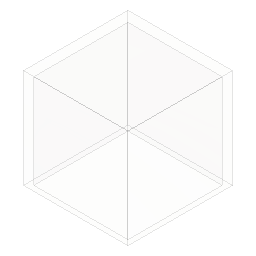
9. Sizing Box (18x18x18in) (Autodesk Fusion 360 design; units mm, degrees)
Autodesk Fusion 360 part; units mm, degrees
sketch "Sketch1" plane through (0, 0, 0) normal (0, 1, 0) x (1, 0, 0)
  line L0 (228.6, -228.6) -> (-228.6, -228.6)
  line L1 (-228.6, -228.6) -> (-228.6, 228.6)
  line L2 (-228.6, 228.6) -> (228.6, 228.6)
  line L3 (228.6, 228.6) -> (228.6, -228.6)
  line L4 (228.6, -228.6) -> (-228.6, 228.6) construction
  line L5 (-228.6, -228.6) -> (228.6, 228.6) construction
  dimension "d1" = 457.2
  dimension "d2" = 457.2
  constraint horizontal L0
  constraint perpendicular L0 L1
  constraint parallel L0 L2
  constraint parallel L1 L3
  constraint coincident L4 origin
  constraint coincident L5 origin
  measures "d1" distance of L1.end L2.end
  measures "d2" distance of L0.end L1.end
extrude "Extrude1" add sketch "Sketch1" along normal blind 457.2 makes body 1
copy_body "Body->Comp1" bodies 1 removing the originals makes body 2 in component "SIzing Box"
delete_body "RemoveBody1" bodies 2 in component "SIzing Box"
sketch "Sketch1 (2)" plane through (0, 0, 0) normal (0, 1, 0) x (1, 0, 0) in component "SIzing Box"
  line L0 (228.6, -228.6) -> (-228.6, -228.6)
  line L1 (-228.6, -228.6) -> (-228.6, 228.6)
  line L2 (-228.6, 228.6) -> (228.6, 228.6)
  line L3 (228.6, 228.6) -> (228.6, -228.6)
  line L4 (228.6, -228.6) -> (-228.6, 228.6) construction
  line L5 (-228.6, -228.6) -> (228.6, 228.6) construction
  line L6 (254, -254) -> (-254, -254)
  line L7 (-254, -254) -> (-254, 254)
  line L8 (-254, 254) -> (254, 254)
  line L9 (254, 254) -> (254, -254)
  dimension "d5" = 457.2
  dimension "d6" = 457.2
  dimension "d7" = -25.4
  constraint horizontal L0
  constraint perpendicular L0 L1
  constraint parallel L0 L2
  constraint parallel L1 L3
  constraint coincident L4 origin
  constraint coincident L5 origin
  measures "d5" distance of L1.end L2.end
  measures "d6" distance of L0.end L1.end
extrude "Extrude2" add sketch "Sketch1 (2)" along normal blind 25.4 from surface at 457.2 separate body contours L0 L1 L2 L3 | L6 L7 L8 L9 makes body 3 in component "SIzing Box"
extrude "Extrude1'" add sketch "Sketch1 (2)" along normal blind 457.2 bodies 3 in component "SIzing Box"
component "SIzing Box" placed x (1, 0, 0) y (0, 1, 0) z (0, 0, 1) at (0, 0, 0)
